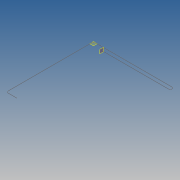
# Autodesk Inventor part: Seil1
Saved by Autodesk Inventor 2015 SP1 (Build 190203100, 203)
## iProperties
Created: 2015-03-05
Part Number: Seil1
Material: Generisch
Document SubType Name: Modeling
Designer: Marc
Mass: 4.44965 g
Surface Area: 89.0557 cm^2
Volume: 4.44965 cm^3
Density: 1 g/cm^3
Appearance: Vorgabe
Author: Marc
Autodesk Inventor part; units mm, degrees
ref_plane "YZ Plane" through (0, 0, 0) normal (1, 0, 0) x (0, 1, 0)
ref_plane "XZ Plane" through (0, 0, 0) normal (0, 1, 0) x (-1, 0, 0)
ref_plane "XY Plane" through (0, 0, 0) normal (0, 0, 1) x (1, 0, 0)
ref_plane "Arbeitsebene1" through (0, 0, 0) normal (0, 0, 1) x (1, 0, 0)
sketch "Skizze5" plane through (0, 0, 0) normal (0, 0, 1) x (1, 0, 0)
  circle A0 centre (0, 0) radius 10 projected
  circle A1 centre (440, 0) radius 10 projected
  line L0 (440, 10) -> (0, 10)
  arc A2 (0, 10) -> (-10, 0) centre (0, 0) ccw
  arc A3 (440, -10) -> (440, 10) centre (440, 0) ccw
  line L1 (440, -10) -> (57.3732, -10)
  circle A4 centre (0, -480) radius 10 projected
  line L2 (-10, 0) -> (-10, -480)
  line L3 (0, -490) -> (50.9075, -490)
  arc A5 (-10, -480) -> (0, -490) centre (0, -480) ccw
  arc A6 (440, -10) -> (440, 10) centre (440, 0) ccw
  point P0 (0, 0)
  constraints: 15 point on circle, 12 tangent, 8 end point, 4 centre point, 2 horizontal, 1 perpendicular
ref_plane "Arbeitsebene4" through (57.3732, -10, 0) normal (-1, 0, 0) x (0, -1, 0)
sketch "Skizze6" plane through (57.3732, -10, 0) normal (-1, 0, 0) x (0, -1, 0)
  circle A0 centre (0, 0) radius 1
  point P0 (-10, 0)
  dimension "d3" = 2
  constraints: 1 centre point, 1 coincident
  measures "d3" diameter of A0
sweep "Sweeping2" add profiles "Skizze6" path "Skizze5" path curves L1 A6 L0 A2 L2 A5 L3
